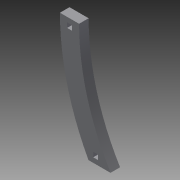
# Autodesk Inventor part: HopperFrontSupport_v1
Saved by Autodesk Inventor 2013 (Build 170138000, 138)
## iProperties
Created: 2013-01-16
Part Number: HopperFrontSupport_v1
Material: Generic
Document SubType Name: Modeling
Designer: twsass
Density: 1 g/cm^3
Author: twsass
Autodesk Inventor part; units mm, degrees
ref_plane "YZ Plane" through (0, 0, 0) normal (1, 0, 0) x (0, 1, 0)
ref_plane "XZ Plane" through (0, 0, 0) normal (0, 1, 0) x (-1, 0, 0)
ref_plane "XY Plane" through (0, 0, 0) normal (0, 0, 1) x (1, 0, 0)
sketch "Sketch1" plane through (0, 0, 0) normal (0, 0, 1) x (1, 0, 0)
  circle A0 centre (0, 0) radius 292.1
  line L0 (-292.1, 0) -> (-266.7, 0)
  line L1 (-292.1, 0) -> (-317.5, 0)
  circle A1 centre (0, 0) radius 317.5
  line L2 (-317.5, 0) -> (-317.5, -150.4188)
  line L3 (-317.5, -150.4188) -> (-250.3929, -150.4188)
  circle A2 centre (0, 0) radius 317.5
  dimension "d0" = 584.2
  dimension "d1" = 25.4
  dimension "d2" = 25.4
  dimension "d3" = 150.4188
  constraints: 8 end point, 3 coincident, 2 centre point, 2 perpendicular, 2 point on circle, 1 collinear, 1 horizontal, 1 horizontal alignment, 1 vertical, 2 other
  measures "d0" diameter of A0
  measures "d1" distance of L0.start L0.end
  measures "d2" distance of L0.start L1.end
  measures "d3" distance of L1.end L2.end
extrude "Extrusion1" add sketch "Sketch1" along normal blind 12.7 contours A0 L3 A1 L1 | A1 L3 L2 picked at (-273.7775, -123.6883)
sketch "Sketch2" plane through (0, 0, 12.7) normal (0, 0, 1) x (1, 0, 0)
  line L0 (-317.5, 0) -> (-317.5, -150.4188) projected
  line L1 (-317.5, -150.4188) -> (-250.3929, -150.4188) projected
  arc A0 (-292.1, 0) -> (-250.3929, -150.4188) centre (0, 0) ccw projected
  circle A1 centre (0, 0) radius 292.1
  circle A2 centre (0, 0) radius 317.5
  line L2 (-317.5, 0) -> (-317.5, -150.4188)
  line L3 (-317.5, -150.4188) -> (-279.6076, -150.4188)
  constraints: 4 end point, 2 centre point, 2 coincident, 2 point on circle, 1 collinear, 1 concentric, 1 point on line, 1 tangent
extrude "Extrusion2" cut sketch "Sketch2" against normal blind 25.4 contours A2 L1 L0
sketch "Sketch3" plane through (0, 0, 12.7) normal (0, 0, 1) x (1, 0, 0)
  arc A0 (-317.5, 0) -> (-279.6076, -150.4188) centre (0, 0) ccw projected
  arc A1 (-292.1, 0) -> (-250.3929, -150.4188) centre (0, 0) ccw projected
  line L0 (-292.1, 0) -> (-317.5, 0) projected
  line L1 (-304.8, 0) -> (-304.8, -6.35)
  line L2 (-304.8, -6.35) -> (-304.8, -12.7)
  line L3 (-304.8, -12.7) -> (-301.625, -12.7)
  line L4 (-301.625, -12.7) -> (-301.625, -6.35)
  line L5 (-301.625, -6.35) -> (-307.975, -6.35)
  line L6 (-307.975, -6.35) -> (-307.975, -12.7)
  line L7 (-307.975, -12.7) -> (-304.8, -12.7)
  line L8 (-279.6076, -150.4188) -> (-304.8, -150.4188)
  line L9 (-284.5263, -140.8938) -> (-284.5263, -150.4188)
  line L10 (-284.5263, -140.8938) -> (-255.8737, -140.8938)
  line L11 (-270.2, -137.7188) -> (-267.025, -137.7188)
  line L12 (-267.025, -137.7188) -> (-267.025, -144.0688)
  line L13 (-267.025, -144.0688) -> (-273.375, -144.0688)
  line L14 (-273.375, -144.0688) -> (-273.375, -137.7188)
  line L15 (-273.375, -137.7188) -> (-270.2, -137.7188)
  dimension "d8" = 6.35
  dimension "d9" = 6.35
  dimension "d10" = 3.175
  dimension "d11" = 6.35
  dimension "d12" = 6.35
  dimension "d14" = 9.525
  dimension "d16" = 3.175
  dimension "d17" = 6.35
  dimension "d18" = 6.35
  dimension "d19" = 3.175
  dimension "d20" = 4.9186
  dimension "d21" = 11.1513
  constraints: 30 end point, 8 perpendicular, 4 parallel, 2 collinear, 2 point on circle, 1 midpoint, 1 point on line
  measures "d8" distance of L1.start L1.end
  measures "d9" distance of L1.end L2.end
  measures "d10" distance of L2.end L3.end
  measures "d11" distance of L3.end L4.end
  measures "d12" distance of L4.end L5.end
  measures "d14" distance of L9.start L9.end
  measures "d16" distance of L11.start L11.end
  measures "d17" distance of L11.end L12.end
  measures "d18" distance of L12.end L13.end
  measures "d19" distance between parallel lines of L10 L15
  measures "d20" distance from line of L8.start L9
  measures "d21" distance from line of L9.start L14
extrude "Extrusion3" cut sketch "Sketch3" against normal blind 25.4 contours L14 L15 L11 L12 L10 | L10 L12 L13 L14 | L5 L4 L3 L2 | L2 L7 L6 L5
body "Solid1"
